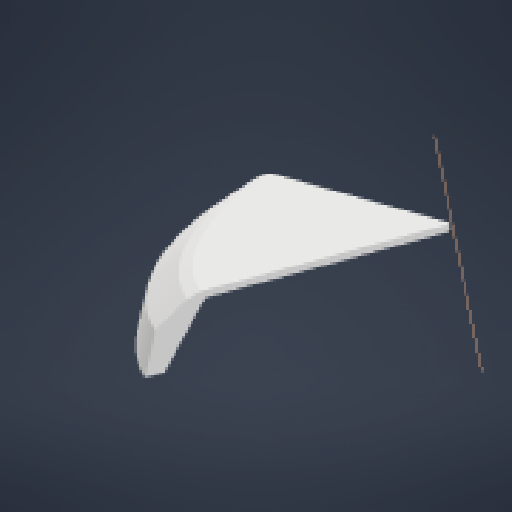
# Autodesk Inventor part: Head_RightPanel_Bottom
Saved by Autodesk Inventor 2024 (Build 280153000, 153)
## iProperties
Created: 2025-09-16
Part Number: Head_RightPanel_Bottom
Material: Generic
Document SubType Name: Modeling
Designer: kevin
Density: 1 g/cm^3
Appearance: Default
Author: kevin
Autodesk Inventor part; units mm, degrees
ref_plane "YZ Plane" through (0, 0, 0) normal (1, 0, 0) x (0, 1, 0)
ref_plane "XZ Plane" through (0, 0, 0) normal (0, 1, 0) x (-1, 0, 0)
ref_plane "XY Plane" through (0, 0, 0) normal (0, 0, 1) x (1, 0, 0)
sketch "Sketch1" plane through (0, 0, 0) normal (0, 0, 1) x (1, 0, 0)
  line L0 (18.7565, 2.6482) -> (25.351, 6.5837) projected
  line L1 (18.7565, 2.6482) -> (3.5965, -13.665) projected
  line L2 (0.3391, -38.6037) -> (3.5965, -13.665) projected
  line L3 (10.018, -36.0901) -> (0.3391, -38.6037) projected
  line L4 (28.0088, 3.1413) -> (10.018, -36.0901) projected
  line L5 (150.5088, 34.9549) -> (28.0088, 3.1413) projected
  line L6 (149.5033, 38.8265) -> (150.5088, 34.9549) projected
  line L7 (25.351, 6.5837) -> (119.9587, 31.1536) projected
  line L8 (152.5414, 35.4828) -> (151.49, 39.5312) construction
  line L9 (119.9587, 31.1536) -> (149.5033, 38.8265) projected
  point P0 (0, 0)
  constraints: 2 end point
revolve "Revolution1" add sketch "Sketch1" angle 60 about axis through (152.5414, 35.4828, 0) along (-0.2514, 0.9679, 0)
body "Solid1"
